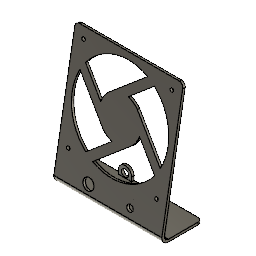
fanStand (Autodesk Fusion 360 design; units mm, degrees)
Autodesk Fusion 360 part; units mm, degrees
sketch "Sketch1" plane through (0, 0, 0) normal (0, 1, 0) x (1, 0, 0)
  line L0 (0, 0) -> (130, 0)
  line L1 (130, 0) -> (130, -145)
  line L2 (125, -150) -> (5, -150)
  line L3 (0, -145) -> (0, 0)
  line L4 (65, -150) -> (65, 0)
  line L5 (0, -20) -> (130, -20)
  line L6 (130, -85) -> (0, -85)
  circle A0 centre (65, -85) radius 57.5
  circle A1 centre (65, -85) radius 25
  line L7 (5, -145) -> (125, -145)
  line L8 (125, -145) -> (125, -25)
  line L9 (125, -25) -> (5, -25)
  line L10 (5, -25) -> (5, -145)
  line L11 (5, -25) -> (12, -32)
  circle A2 centre (12, -32) radius 2
  line L12 (125, -25) -> (118, -32)
  circle A3 centre (118, -32) radius 2
  line L13 (125, -145) -> (118, -138)
  circle A4 centre (118, -138) radius 2
  line L14 (5, -145) -> (12, -138)
  circle A5 centre (12, -138) radius 2
  line L15 (65, -85) -> (82.6777, -102.6777)
  line L16 (65, -85) -> (90, -85) construction
  line L17 (65, -85) -> (82.6777, -67.3223)
  line L18 (65, -85) -> (90, -85) construction
  line L19 (65, -85) -> (47.3223, -102.6777)
  line L20 (65, -85) -> (90, -85) construction
  line L21 (65, -85) -> (47.3223, -67.3223)
  line L22 (65, -85) -> (90, -85) construction
  line L23 (82.6777, -67.3223) -> (32.2399, -25)
  line L24 (82.6777, -67.3223) -> (148.5195, -67.3223) construction
  line L25 (82.6777, -102.6777) -> (125, -52.2399)
  line L26 (82.6777, -102.6777) -> (148.5195, -102.6777) construction
  line L27 (47.3223, -102.6777) -> (97.7601, -145)
  line L28 (47.3223, -67.3223) -> (0, -123.7189)
  circle A6 centre (40, -10) radius 6.5
  circle A7 centre (90, -10) radius 3.75
  arc A8 (0, -145) -> (5, -150) centre (5, -145) ccw
  arc A9 (125, -150) -> (130, -145) centre (125, -145) ccw
  line L29 (47.3223, -67.3223) -> (5, -117.7601)
  line L30 (5, -117.7601) -> (12.6604, -124.188)
  line L31 (12.6604, -124.188) -> (54.9828, -73.7502)
  line L32 (54.9828, -73.7502) -> (47.3223, -67.3223)
  line L33 (47.3223, -102.6777) -> (97.7601, -145)
  line L34 (97.7601, -145) -> (104.188, -137.3396)
  line L35 (104.188, -137.3396) -> (53.7502, -95.0172)
  line L36 (53.7502, -95.0172) -> (47.3223, -102.6777)
  line L37 (82.6777, -102.6777) -> (125, -52.2399)
  line L38 (125, -52.2399) -> (117.3396, -45.812)
  line L39 (117.3396, -45.812) -> (75.0172, -96.2498)
  line L40 (75.0172, -96.2498) -> (82.6777, -102.6777)
  line L41 (82.6777, -67.3223) -> (32.2399, -25)
  line L42 (32.2399, -25) -> (25.812, -32.6604)
  line L43 (25.812, -32.6604) -> (76.2498, -74.9828)
  line L44 (76.2498, -74.9828) -> (82.6777, -67.3223)
  dimension "d1" = 50
  dimension "d2" = 115
  dimension "d3" = 45
  dimension "d4" = 45
  dimension "d5" = 135
  dimension "d6" = 135
  dimension "d7" = 140
  dimension "d8" = 50
  dimension "d9" = 13
  dimension "d10" = 7.5
  dimension "d11" = 5
  dimension "d12" = 5
  dimension "d13" = 10
  dimension "d14" = 10
  dimension "d15" = 10
  dimension "d16" = 10
  constraint horizontal L0
  constraint vertical L1
  constraint horizontal L2
  constraint vertical L3
  constraint coincident L0.start L3.end
  constraint midpoint L0 L4.end
  constraint coincident L3 L5.start
  constraint coincident L1 L5.end
  constraint perpendicular L1 L5
  constraint coincident L1 L6.start
  constraint coincident L3 L6.end
  constraint perpendicular L3 L6
  constraint midpoint L6 A0.centre
  constraint concentric A0 A1
  constraint horizontal L7
  constraint vertical L8
  constraint horizontal L9
  constraint vertical L10
  constraint coincident L11.end A2.centre
  constraint coincident L12.end A3.centre
  constraint coincident L13.end A4.centre
  constraint coincident L14.end A5.centre
  constraint horizontal L16
  constraint coincident A0.centre A1.centre
  constraint horizontal L18
  constraint horizontal L20
  constraint horizontal L22
  constraint horizontal L24
  constraint coincident L9 L23.end
  constraint horizontal L26
  constraint coincident L8 L25.end
  constraint coincident L7 L27.end
  constraint perpendicular L25 L27
  constraint perpendicular L27 L28
  constraint coincident L2 L4.start
  constraint tangent L2 A8
  constraint tangent L3 A8
  constraint tangent L1 A9
  constraint tangent L2 A9
  constraint coincident L3 L28.end
  constraint coincident L7.start L10
  constraint perpendicular L29 L30
  constraint parallel L29 L31
  constraint parallel L30 L32
  constraint coincident L10 L29.end
  constraint coincident L28 L29.end
  constraint perpendicular L33 L34
  constraint parallel L33 L35
  constraint parallel L34 L36
  constraint parallel L27 L33
  constraint perpendicular L37 L38
  constraint parallel L37 L39
  constraint parallel L38 L40
  constraint parallel L25 L37
  constraint perpendicular L41 L42
  constraint parallel L41 L43
  constraint parallel L42 L44
  constraint parallel L23 L41
  measures "d1" diameter of A1
  measures "d2" diameter of A0
  measures "d3" angle of L15 L16
  measures "d4" angle of L17 L18
  measures "d5" angle of L19 L20
  measures "d6" angle of L21 L22
  measures "d7" angle of L23 L24
  measures "d8" angle of L25 L26
  measures "d9" diameter of A6
  measures "d10" diameter of A7
  measures "d11" radius of A8
  measures "d12" radius of A9
  measures "d13" distance of L21.end L31.end
  measures "d14" distance of L19.end L35.end
  measures "d15" distance of L15.end L39.end
  measures "d16" distance of L17.end L43.end
extrude "Extrude1" add sketch "Sketch1" along normal blind 3 contours L0 L3 L4 L5 | L0 L1 L4 L5 | L3 L4 L5 L6 L9 L10 | L1 L4 L5 L6 L8 L9 | L3 L6 L10 L28 | L4 A0 L8 L9 L38 L39 | L4 A0 L9 L23 L41 | L2 L3 L4 L7 L10 L28 A8 | L6 A0 L9 L10 L42 L43 | L6 A0 L10 L28 L29 | L1 L2 L4 L6 L7 L8 A9 | A0 L23 L41 L42 L43 | L4 A0 L7 L10 L30 L31 | A0 L28 L29 L30 L31 | L6 A0 L7 L8 L34 L35 | L6 A0 L8 L25 L37 | L4 A1 L23 L41 | L4 A0 A1 L23 L41 L43 | A0 L25 L37 L38 L39 | L6 A0 A1 L25 L37 L39 | L6 A0 A1 L28 L29 L31 | L6 A1 L28 L29 | L4 A1 L17 L23 L41 L43 | L4 A1 L43 | L6 A1 L17 L39 L43 L44 | L6 A1 L39 | L4 A0 L7 L27 L33 | L6 A1 L21 L28 L29 L31 | L6 A1 L31 | L4 A1 L21 L31 L32 L43 | L6 A1 L25 L37 | A0 L27 L33 L34 L35 | L4 A0 A1 L27 L33 L35 | L4 L17 L43 | L17 L43 L44 | L6 A1 L15 L25 L37 L39 | L6 L15 L39 | L6 A1 L19 L31 L35 L36 | L6 L21 L31 | L21 L31 L32 | L4 A1 L15 L35 L39 L40 | L4 A1 L35 | L4 L19 L35 | L15 L39 L40 | L4 A1 L27 L33 | L19 L35 L36 | L4 A1 L19 L27 L33 L35
sketch "Sketch2" plane through (0, 3, 0) normal (0, 1, 0) x (-1, 0, 0)
  circle A0 centre (-118, 138) radius 2
  arc A1 (-17.8852, 117.9613) -> (-88.6929, 137.3917) centre (-65, 85) ccw
  line L0 (-17.8852, 117.9613) -> (-40.6808, 90.7946)
  arc A2 (-40.6808, 90.7946) -> (-47.3223, 102.6777) centre (-65, 85) ccw
  line L1 (-47.3223, 102.6777) -> (-88.6929, 137.3917)
  circle A3 centre (-12, 32) radius 2
  circle A4 centre (-12, 138) radius 2
  circle A5 centre (-90, 10) radius 3.75
  circle A6 centre (-40, 10) radius 6.5
  circle A7 centre (-118, 32) radius 2
  line L2 (-32.0387, 37.8852) -> (-59.2054, 60.6808)
  arc A8 (-59.2054, 60.6808) -> (-47.3223, 67.3223) centre (-65, 85) ccw
  line L3 (-47.3223, 67.3223) -> (-12.6083, 108.6929)
  arc A9 (-32.0387, 37.8852) -> (-12.6083, 108.6929) centre (-65, 85) ccw
  arc A10 (-112.1148, 52.0387) -> (-41.3071, 32.6083) centre (-65, 85) ccw
  line L4 (-112.1148, 52.0387) -> (-89.3192, 79.2054)
  arc A11 (-89.3192, 79.2054) -> (-82.6777, 67.3223) centre (-65, 85) ccw
  line L5 (-82.6777, 67.3223) -> (-41.3071, 32.6083)
  arc A12 (-97.9613, 132.1148) -> (-117.3917, 61.3071) centre (-65, 85) ccw
  line L6 (-97.9613, 132.1148) -> (-70.7946, 109.3192)
  arc A13 (-70.7946, 109.3192) -> (-82.6777, 102.6777) centre (-65, 85) ccw
  line L7 (-82.6777, 102.6777) -> (-117.3917, 61.3071)
  arc A14 (0, 145) -> (-5, 150) centre (-5, 145) ccw
  line L8 (-5, 150) -> (-125, 150)
  arc A15 (-125, 150) -> (-130, 145) centre (-125, 145) ccw
  line L9 (-130, 145) -> (-130, 0)
  line L10 (-130, 0) -> (0, 0)
  line L11 (0, 0) -> (0, 145)
move_body "Move1" bodies 1 to x (1, 0, 0) y (0, 0.984808, -0.173648) z (0, 0.173648, 0.984808) at (0, 0.0456, 0.5209)
sketch "Sketch3" plane through (130, 0, 0) normal (1, 0, 0) x (0, 1, 0)
  line L0 (25.2246, 143.3181) -> (0.0456, 0.5209)
  line L1 (0.0456, 0.5209) -> (3, 0)
  line L2 (3, 0) -> (28.179, 142.7971)
  line L3 (28.179, 142.7971) -> (25.2246, 143.3181)
  line L4 (7, 0) -> (3, 0) construction
  line L5 (28.179, 142.7971) -> (54.4361, 136.5073)
  line L6 (54.4361, 136.5073) -> (54.4361, -10)
  line L7 (3, 0) -> (8, 0)
  line L8 (8, 0) -> (8, -11)
  arc A0 (3, 0) -> (8, -5) centre (8, 0) ccw
  arc A1 (0.0456, 0.5209) -> (8, -7.9715) centre (8, 0) ccw
  line L9 (8, -5) -> (54.4361, -5)
  line L10 (8, -7.9715) -> (55, -7.9715)
  dimension "d21" = 27
  constraint coincident L1.end L2.start
  constraint coincident L2.end L3.start
  constraint vertical L6
  constraint parallel L4 L7
  constraint perpendicular L7 L8
  constraint coincident L8 A0.end
  constraint coincident L7.end L8.start
  constraint coincident L8 A1.end
  constraint coincident L0.end L1.start
  constraint coincident L6 L9.end
  constraint perpendicular L6 L9
  constraint tangent A1 L10
  constraint perpendicular L6 L10
  measures "d21" distance of L2.end L5.end
extrude "Extrude2" add sketch "Sketch3" against normal blind 130 contours L1 L8 A0 A1 | L6 L8 L9 L10
sketch "Sketch4" plane through (0, 0, 0) normal (-1, 0, 0) x (0, -1, 0)
  line L0 (-0.0456, 0.5209) -> (-25.2246, 143.3181)
  line L1 (-25.2246, 143.3181) -> (-28.179, 142.7971)
  line L2 (-28.179, 142.7971) -> (-3, 0)
  arc A0 (-8, -5) -> (-3, 0) centre (-8, 0) ccw
  line L3 (-8, -5) -> (-54.4361, -5)
  line L4 (-54.4361, -5) -> (-54.4361, -7.9715)
  line L5 (-54.4361, -7.9715) -> (-8, -7.9715)
  arc A1 (-8, -7.9715) -> (-0.0456, 0.5209) centre (-8, 0) ccw
  circle A2 centre (-11, 2) radius 4
  line L6 (-11, 2) -> (-17, 8)
  arc A3 (-17, 8) -> (-15.7958, -5) centre (-11, 2) ccw
  arc A4 (-4.2621, 7.1575) -> (-17, 8) centre (-11, 2) ccw
  line L7 (-11, 10.4853) -> (-4.8488, 10.4853)
  line L8 (-19.4853, 2) -> (-19.4853, -5)
  line L9 (-17, 8) -> (-6.2977, 18.7023)
  constraint coincident A2.centre L6.start
  constraint coincident L3 A3.end
  constraint coincident L2 A4.start
  constraint coincident A4 L7.start
  constraint coincident L2 L7.end
  constraint tangent A4 L7
  constraint horizontal L7
  constraint coincident A3 L8.start
  constraint coincident L3 L8.end
  constraint tangent A3 L8
  constraint perpendicular L3 L8
  constraint coincident L2 L9.end
  constraint tangent A4 L9
sketch "Sketch5" plane through (0, 0, -5) normal (0, 0, 1) x (-1, 0, 0)
  line L0 (0, -8) -> (-130, -8)
  line L1 (-130, -8) -> (-130, -54.4361)
  line L2 (-130, -54.4361) -> (0, -54.4361)
  line L3 (0, -54.4361) -> (0, -8)
  line L4 (0, -43.6935) -> (0, -31.2181)
  line L5 (-5, -48.6935) -> (-125, -48.6935)
  line L6 (-130, -43.6935) -> (-130, -31.2181)
  arc A0 (-5, -48.6935) -> (0, -43.6935) centre (-5, -43.6935) ccw
  arc A1 (-130, -43.6935) -> (-125, -48.6935) centre (-125, -43.6935) ccw
  dimension "d26" = 5
  dimension "d27" = 5
  constraint midpoint L3 L4.end
  constraint midpoint L1 L6.end
  constraint tangent L4 A0
  constraint tangent L5 A0
  constraint tangent L6 A1
  constraint tangent L5 A1
  measures "d26" radius of A0
  measures "d27" radius of A1
extrude "Extrude4" cut sketch "Sketch5" against normal blind 3 contours L1 L2 L3 L5 A0 A1
sketch "Sketch7" plane through (0, 48.6935, 0) normal (0, 1, 0) x (-1, 0, 0)
  line L0 (-125, -7.9715) -> (-5, -7.9715)
  line L1 (-5, -7.9715) -> (-5, -5)
  line L2 (-5, -5) -> (-125, -5)
  line L3 (-125, -5) -> (-125, -7.9715)
  circle A0 centre (-40, 0) radius 4.25
  circle A1 centre (-40, 0) radius 8
  line L4 (-32, 0) -> (-32, -5)
  line L5 (-48, 0) -> (-48, -5)
  dimension "d30" = 8.5
  constraint concentric A0 A1
  constraint coincident A1 L4.start
  constraint coincident L2 L4.end
  constraint tangent A1 L4
  constraint perpendicular L2 L4
  constraint coincident A1 L5.start
  constraint coincident L2 L5.end
  constraint tangent A1 L5
  constraint perpendicular L2 L5
  measures "d30" diameter of A0
extrude "Extrude5" add sketch "Sketch7" against normal blind 3 contours L2 A1 | L2 A1 L5 | L2 A1 L4
sketch "Sketch8" plane through (0, 2.9095, -0.513) normal (0, 0.984808, -0.173648) x (-1, 0, 0)
  circle A0 centre (-118, 138.5209) radius 2
  arc A1 (-17.8852, 118.4823) -> (-88.6929, 137.9127) centre (-65, 85.5209) ccw
  line L0 (-17.8852, 118.4823) -> (-40.6808, 91.3156)
  arc A2 (-40.6808, 91.3156) -> (-47.3223, 103.1986) centre (-65, 85.5209) ccw
  line L1 (-47.3223, 103.1986) -> (-88.6929, 137.9127)
  circle A3 centre (-12, 32.5209) radius 2
  circle A4 centre (-12, 138.5209) radius 2
  circle A5 centre (-90, 10.5209) radius 3.75
  circle A6 centre (-40, 10.5209) radius 6.5
  circle A7 centre (-118, 32.5209) radius 2
  line L2 (-32.0387, 38.4062) -> (-59.2054, 61.2018)
  arc A8 (-59.2054, 61.2018) -> (-47.3223, 67.8433) centre (-65, 85.5209) ccw
  line L3 (-47.3223, 67.8433) -> (-12.6083, 109.2139)
  arc A9 (-32.0387, 38.4062) -> (-12.6083, 109.2139) centre (-65, 85.5209) ccw
  arc A10 (-112.1148, 52.5596) -> (-41.3071, 33.1292) centre (-65, 85.5209) ccw
  line L4 (-112.1148, 52.5596) -> (-89.3192, 79.7263)
  arc A11 (-89.3192, 79.7263) -> (-82.6777, 67.8433) centre (-65, 85.5209) ccw
  line L5 (-82.6777, 67.8433) -> (-41.3071, 33.1292)
  arc A12 (-97.9613, 132.6357) -> (-117.3917, 61.828) centre (-65, 85.5209) ccw
  line L6 (-97.9613, 132.6357) -> (-70.7946, 109.8401)
  arc A13 (-70.7946, 109.8401) -> (-82.6777, 103.1986) centre (-65, 85.5209) ccw
  line L7 (-82.6777, 103.1986) -> (-117.3917, 61.828)
  arc A14 (0, 145.5209) -> (-5, 150.5209) centre (-5, 145.5209) ccw
  line L8 (-5, 150.5209) -> (-125, 150.5209)
  arc A15 (-125, 150.5209) -> (-130, 145.5209) centre (-125, 145.5209) ccw
  line L9 (-130, 145.5209) -> (-130, 0.5209)
  line L10 (-130, 0.5209) -> (0, 0.5209)
  line L11 (0, 0.5209) -> (0, 145.5209)
  line L12 (-90, 10.5209) -> (-90, 18.5209)
  line L13 (-88, 17.5209) -> (-92, 17.5209)
  line L14 (-92, 17.5209) -> (-92, 19.5209)
  line L15 (-92, 19.5209) -> (-88, 19.5209)
  line L16 (-88, 19.5209) -> (-88, 17.5209)
  line L17 (-88, 17.5209) -> (-92, 19.5209) construction
  line L18 (-92, 17.5209) -> (-88, 19.5209) construction
  line L19 (-90, 10.5209) -> (-97, 10.5209)
  line L20 (-92, 3.5209) -> (-92, 1.5209)
  line L21 (-88, 3.5209) -> (-92, 3.5209)
  line L22 (-88, 1.5209) -> (-88, 3.5209)
  line L23 (-92, 1.5209) -> (-88, 1.5209)
  point P0 (-90, 18.5209)
  point P1 (-90, 10.5209)
  dimension "d35" = 2
  dimension "d36" = 4
  dimension "d37" = 8
  constraint coincident P1 A5.centre
  constraint vertical L12
  constraint perpendicular L13 L14
  constraint parallel L13 L15
  constraint parallel L14 L16
  constraint horizontal L13
  constraint coincident L17 P0
  constraint coincident L18 P0
  constraint coincident P0 L12.end
  constraint perpendicular L12 L19
  constraint symmetric P1 L19 A5.centre
  constraint symmetric L13.start L19 L21.start
  constraint symmetric L13.end L19 L20.start
  constraint symmetric L14.end L19 L20.end
  constraint symmetric L15.end L19 L22.start
  measures "d35" distance of L13.end L14.end
  measures "d36" distance of L13.start L13.end
  measures "d37" distance of P1 P0
extrude "Extrude6" cut sketch "Sketch8" against normal blind 2 contours L13 L14 L15 L16 | L20 L21 L22 L23
